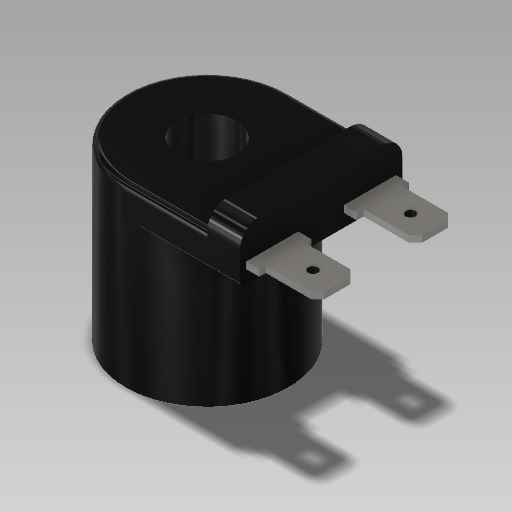
# Autodesk Inventor part: Solenoide
Saved by Autodesk Inventor 2020 (Build 240168000, 168)
## iProperties
Created: 2019-04-28
Part Number: Solenoide
Material: Generic
Document SubType Name: Modeling
Designer: Plo
Density: 1 g/cm^3
Appearance: Glossy - Black
Author: Plo
Autodesk Inventor part; units mm, degrees
ref_plane "XZ Plane" through (0, 0, 0) normal (0, 1, 0) x (-1, 0, 0)
ref_plane "XY Plane" through (0, 0, 0) normal (0, 0, 1) x (1, 0, 0)
sketch "Sketch1" plane through (0, 0, 0) normal (0, 1, 0) x (-1, 0, 0)
  circle A0 centre (0, 0) radius 12.5
  dimension "d0" = 25
  constraints: 1 centre point, 1 coincident
  measures "d0" diameter of A0
extrude "Extrusion1" add sketch "Sketch1" along normal blind 27
ref_plane "Work Plane1" through (12.5, 0, 0) normal (1, 0, 0) x (0, 1, 0)
sketch "Sketch2" plane through (12.5, 0, 0) normal (1, 0, 0) x (0, 1, 0)
  line L0 (27, -12.5) -> (27, 12.5) projected
  line L1 (27, 12.5) -> (27, -12.5)
  line L2 (27, -12.5) -> (22, -12.5)
  line L3 (0, -12.5) -> (27, -12.5) projected
  line L4 (22, -12.5) -> (22, 12.5)
  line L5 (22, 12.5) -> (27, 12.5)
  line L6 (0, 12.5) -> (27, 12.5) projected
  point P0 (0, 0)
  dimension "d3" = 5
  constraints: 8 end point, 2 collinear, 1 point on line, 1 vertical
  measures "d3" distance of L0.start L2.end
extrude "Extrusion2" add sketch "Sketch2" against normal up to next
sketch "Sketch3" plane through (12.5, 0, 0) normal (1, 0, 0) x (0, 0, -1)
  line L0 (-12.5, 22) -> (-12.5, 27) projected
  line L1 (-12.5, 22) -> (-12.5, 30)
  line L2 (-12.5, 30) -> (12.5, 30)
  line L3 (12.5, 22) -> (12.5, 27) projected
  line L4 (12.5, 30) -> (12.5, 22)
  line L5 (-12.5, 22) -> (0, 22) projected
  line L6 (12.5, 22) -> (-12.5, 22)
  point P0 (0, 0)
  dimension "d6" = 8
  constraints: 8 end point, 2 collinear, 1 perpendicular, 1 vertical
  measures "d6" distance of L0.start L1.end
extrude "Extrusion3" add sketch "Sketch3" along normal blind 5
sketch "Sketch4" plane through (17.5, 0, 0) normal (1, 0, 0) x (0, 0, -1)
  line L0 (-12.5, 22) -> (12.5, 22) projected
  line L1 (-12.5, 22) -> (-12.5, 24)
  line L2 (-12.5, 24) -> (-11.5, 24)
  line L3 (-11.5, 24) -> (-11.5, 25)
  line L4 (-11.5, 25) -> (-3.5, 25)
  line L5 (-3.5, 25) -> (-3.5, 24)
  line L6 (-3.5, 24) -> (-11.5, 24)
  point P0 (0, 0)
  dimension "d9" = 2
  dimension "d10" = 1
  dimension "d11" = 1
  dimension "d12" = 8
  dimension "d13" = 1
  constraints: 12 end point, 3 perpendicular, 1 point on line, 1 vertical
  measures "d9" distance of L0.start L1.end
  measures "d10" distance of L1.end L2.end
  measures "d11" distance of L2.end L3.end
  measures "d12" distance of L3.end L4.end
  measures "d13" distance of L4.end L5.end
extrude "Extrusion4" add sketch "Sketch4" along normal blind 10
sketch "Sketch5" plane through (17.5, 25, 11.5) normal (0, 1, 0) x (1, 0, 0)
  line L0 (10, 0) -> (10, 8) projected
  line L1 (10, 4) -> (6.25, 4)
  circle A0 centre (6.25, 4) radius 0.75
  line L2 (0, 8) -> (10, 8) projected
  line L3 (10, 8) -> (10, 7)
  line L4 (9, 7) -> (2, 7)
  line L5 (2, 7) -> (2, 8)
  line L6 (0, 8) -> (10, 8) projected
  line L7 (10, 7) -> (10, 6)
  line L8 (9, 7) -> (10, 6)
  line L9 (9, 1) -> (2, 1)
  line L10 (2, 1) -> (2, 0)
  line L11 (9, 1) -> (10, 2)
  line L12 (0, 0) -> (10, 0) projected
  line L13 (2, 0) -> (10, 0)
  line L14 (10, 0) -> (10, 2)
  point P0 (-17.5, 11.5)
  constraints: 22 end point, 4 symmetric about line, 3 perpendicular, 3 point on line, 2 horizontal, 1 centre point, 1 coincident, 1 midpoint
extrude "Extrusion5" cut sketch "Sketch5" against normal up to next
mirror "Mirror1" about plane through (0, 0, 0) normal (0, 0, 1) of "Extrusion4", "Extrusion5"
fillet "Fillet1" radius 3 2 edges at (15, 30, 12.5) (15, 30, -12.5)
fillet "Fillet1" radius 1 6 edges at (8.75, 22, -12.5) (-8.8388, 27, 8.8388) (-8.8388, 27, -8.8388) (6.25, 27, 12.5) (6.25, 27, -12.5) (8.75, 22, 12.5)
sketch "Sketch6" plane through (0, 0, 0) normal (0, -1, 0) x (1, 0, 0)
  circle A0 centre (0, 0) radius 4.5
  dimension "d26" = 9
  constraints: 1 centre point, 1 coincident
  measures "d26" diameter of A0
extrude "Extrusion6" cut sketch "Sketch6" against normal up to next
body "Solid1"
